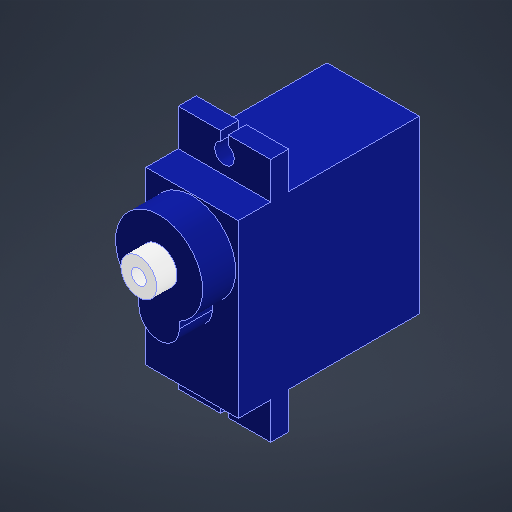
# Autodesk Inventor part: SG90 Servo
Saved by Autodesk Inventor 2025.1 (Build 291241000, 241)
## iProperties
Created: 2024-10-27
Part Number: SG90 Servo
Material: Generic
Document SubType Name: Modeling
Designer: jerem
Density: 1 g/cm^3
Appearance: Default
Author: jerem
Autodesk Inventor part; units mm, degrees
ref_plane "YZ Plane" through (0, 0, 0) normal (1, 0, 0) x (0, 1, 0)
ref_plane "XZ Plane" through (0, 0, 0) normal (0, 1, 0) x (-1, 0, 0)
ref_plane "XY Plane" through (0, 0, 0) normal (0, 0, 1) x (1, 0, 0)
sketch "Sketch1" plane through (0, 0, 0) normal (0, 0, 1) x (1, 0, 0)
  line L0 (6.15, -11.4) -> (-6.15, -11.4)
  line L1 (-6.15, -11.4) -> (-6.15, 11.4)
  line L2 (-6.15, 11.4) -> (6.15, 11.4)
  line L3 (6.15, 11.4) -> (6.15, -11.4)
  line L4 (6.15, -11.4) -> (-6.15, 11.4) construction
  line L5 (-6.15, -11.4) -> (6.15, 11.4) construction
  line L6 (-6.15, 11.4) -> (-6.15, 16.3)
  line L7 (6.15, 16.3) -> (6.15, 11.4)
  line L8 (-6.15, -11.4) -> (-6.15, -16.3)
  line L9 (6.15, -16.3) -> (6.15, -11.4)
  arc A0 (-0.5, 15.1) -> (0.5, 15.1) centre (0, 13.9) ccw
  line L10 (0, 13.9) -> (0, 11.4) construction
  line L11 (-0.5, 16.3) -> (-0.5, 15.1)
  line L12 (0.5, 15.1) -> (0.5, 16.3)
  line L13 (-0.5, 15.1) -> (0.5, 15.1) construction
  line L14 (0, 13.9) -> (0, 15.1) construction
  line L15 (-6.15, 16.3) -> (-0.5, 16.3)
  line L16 (0.5, 16.3) -> (6.15, 16.3)
  arc A1 (0.5, -15.1) -> (-0.5, -15.1) centre (0, -13.9) ccw
  line L17 (-0.5, -15.1) -> (-0.5, -16.3)
  line L18 (0.5, -15.1) -> (0.5, -16.3)
  line L19 (-0.5, -15.1) -> (0.5, -15.1) construction
  line L20 (0, -15.1) -> (0, -13.9) construction
  line L21 (0, -13.9) -> (0, -11.4) construction
  line L22 (-6.15, -16.3) -> (-0.5, -16.3)
  line L23 (0.5, -16.3) -> (6.15, -16.3)
  line L24 (0, 11.4) -> (0, 5.4) construction
  circle A2 centre (0, 5.4) radius 1
  circle A3 centre (0, 5.4) radius 2.4
  arc A4 (-2.7, -0.6) -> (2.7, -0.6) centre (0, -0.6) ccw
  line L25 (0, 5.4) -> (0, -0.6) construction
  line L26 (-2.7, -0.6) -> (-2.7, 0.2668)
  line L27 (2.7, -0.6) -> (2.7, 0.2668)
  arc A5 (2.7, 0.2668) -> (-2.7, 0.2668) centre (0, 5.4) ccw
  point P0 (0, 0)
  dimension "d0" = 22.8
  dimension "d1" = 12.3
  dimension "d4" = 2.6
  dimension "d5" = 2.5
  dimension "d6" = 1
  dimension "d7" = 4.9
  dimension "d8" = 2.5
  dimension "d9" = 1
  dimension "d10" = 2.6
  dimension "d11" = 4.9
  dimension "d14" = 6
  dimension "d15" = 2
  dimension "d16" = 4.8
  dimension "d17" = 5.4
  dimension "d18" = 6
  dimension "d19" = 5.8
  constraints: 57 end point, 15 perpendicular, 10 vertical, 8 point on circle, 6 centre point, 6 midpoint, 3 horizontal, 3 parallel, 2 coincident, 2 collinear, 2 tangent
  measures "d0" distance of L0.end L1.end
  measures "d1" distance of L1.end L2.end
  measures "d4" diameter of A0
  measures "d5" distance of L10.start L10.end
  measures "d6" distance between parallel lines of L12 L11
  measures "d7" distance between parallel lines of L2 L16
  measures "d8" distance of L20.end L21.end
  measures "d9" distance between parallel lines of L18 L17
  measures "d10" diameter of A1
  measures "d11" distance between parallel lines of L0 L23
  measures "d14" distance of L10.end L24.end
  measures "d15" diameter of A2
  measures "d16" diameter of A3
  measures "d17" diameter of A4
  measures "d18" distance of L25.start L25.end
  measures "d19" radius of A5
extrude "Extrusion1" add sketch "Sketch1" against normal blind 17.4 contours L0 L1 L2 L3 | A2 | A3 | L26 A5 L27 A4
extrude "Extrusion2" add sketch "Sketch1" along normal blind 2.4 contours L9 L23 L18 A1 L17 L22 L8 L0 | L0 L1 L2 L3 | L2 L6 L15 L11 A0 L12 L16 L7 | A2 | A3 | L26 A5 L27 A4
extrude "Extrusion3" add sketch "Sketch1" along normal blind 4.3 from surface at 2.4 contours L0 L1 L2 L3 | A2 | A3 | L26 A5 L27 A4
extrude "Extrusion4" add sketch "Sketch1" along normal blind 4.4 from surface at 6.7 contours A2 | A3 | L26 A5 L27 A4
extrude "Extrusion5" add sketch "Sketch1" along normal blind 2.7 from surface at 11.1 contours A3
equation "\"d8\" = d5"
equation "\"d9\" = d6"
equation "\"d10\" = d4"
equation "\"d11\" = d7"
equation "\"d3\" = d2"
equation "\"d2\" = 4.9"
body "Solid1"
